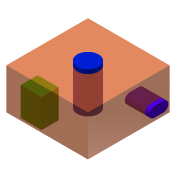
# Autodesk Inventor part: Remnant3Features
Saved by Autodesk Inventor 2014 (Build 180170000, 170)
## iProperties
Created: 2015-06-22
Part Number: Remnant3Features
Material: Generic
Document SubType Name: Modeling
Designer: kulkarni
Density: 1 g/cm^3
Appearance: Default
Author: kulkarni
Autodesk Inventor part; units mm, degrees
ref_plane "YZ Plane" through (0, 0, 0) normal (1, 0, 0) x (0, 1, 0)
ref_plane "XZ Plane" through (0, 0, 0) normal (0, 1, 0) x (-1, 0, 0)
ref_plane "XY Plane" through (0, 0, 0) normal (0, 0, 1) x (1, 0, 0)
sketch "Sketch1" plane through (0, 0, 0) normal (0, 1, 0) x (-1, 0, 0)
  line L0 (0, 0) -> (25.4, 0)
  line L1 (25.4, 0) -> (25.4, -25.4)
  line L2 (25.4, -25.4) -> (0, -25.4)
  line L3 (0, -25.4) -> (0, 0)
  dimension "d0" = 25.4
  dimension "d1" = 25.4
  constraints: 8 end point, 2 parallel, 1 horizontal, 1 perpendicular
  measures "d0" distance of L1.end L2.end
  measures "d1" distance of L0.end L1.end
extrude "Extrusion1" add sketch "Sketch1" along normal blind 12.7
sketch "Sketch2" plane through (0, 12.7, 0) normal (0, 1, 0) x (1, 0, 0)
  circle A0 centre (-12.7, 12.7) radius 3.3294
  constraints: 1 centre point
extrude "Extrusion2" add sketch "Sketch2" along normal blind 1.27 and the other way blind 11.43 separate body
sketch "Sketch3" plane through (0, 0, 0) normal (0, -1, 0) x (1, 0, 0)
  line L0 (-22.9422, -1.9615) -> (-16.3998, -1.9615)
  line L1 (-16.3998, -1.9615) -> (-16.3998, -7.2405)
  line L2 (-16.3998, -7.2405) -> (-22.9422, -7.2405)
  line L3 (-22.9422, -7.2405) -> (-22.9422, -1.9615)
  constraints: 8 end point, 2 parallel, 1 horizontal, 1 perpendicular
extrude "Extrusion3" add sketch "Sketch3" along normal blind 1.27 and the other way blind 7.62 separate body
sketch "Sketch4" plane through (0, 0, 0) normal (1, 0, 0) x (0, 0, -1)
  line L0 (25.4, 0) -> (0, 0) projected
  line L1 (19.3778, 3.733) -> (22.2203, 3.733) construction
  line L2 (19.3778, 2.1792) -> (22.2203, 2.1792)
  line L3 (22.2203, 5.2869) -> (19.3778, 5.2869)
  arc A0 (19.3778, 5.2869) -> (19.3778, 2.1792) centre (19.3778, 3.733) ccw
  arc A1 (22.2203, 2.1792) -> (22.2203, 5.2869) centre (22.2203, 3.733) ccw
  point P0 (20.799, 3.733)
  constraints: 8 end point, 4 point on circle, 4 tangent, 2 centre point, 2 parallel, 1 midpoint
extrude "Extrusion4" add sketch "Sketch4" along normal blind 1.27 and the other way blind 6.35 separate body
body "Solid1"
body "Solid2"
body "Solid3"
body "Solid4"
